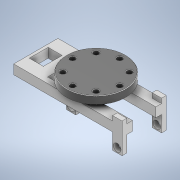
# Autodesk Inventor part: KukaHead
Saved by Autodesk Inventor 2021 (Build 250183000, 183)
## iProperties
Created: 2021-06-08
Part Number: KukaHead
Material: Generic
Document SubType Name: Modeling
Designer: zmac845
Density: 1 g/cm^3
Appearance: Default
Author: zmac845
Autodesk Inventor part; units mm, degrees
ref_plane "YZ Plane" through (0, 0, 0) normal (1, 0, 0) x (0, 1, 0)
ref_plane "XZ Plane" through (0, 0, 0) normal (0, 1, 0) x (-1, 0, 0)
ref_plane "XY Plane" through (0, 0, 0) normal (0, 0, 1) x (1, 0, 0)
sketch "Sketch1" plane through (0, 0, 0) normal (0, 1, 0) x (-1, 0, 0)
  circle A0 centre (0, 0) radius 31.25
  circle A1 centre (0, 25) radius 2.75
  circle A2 centre (-17.6777, 17.6777) radius 2.75
  circle A3 centre (-25, 0) radius 2.75
  circle A4 centre (-17.6777, -17.6777) radius 2.75
  circle A5 centre (0, -25) radius 2.75
  circle A6 centre (17.6777, -17.6777) radius 2.75
  circle A7 centre (25, 0) radius 2.75
  circle A8 centre (17.6777, 17.6777) radius 2.75
  dimension "d0" = 62.5
  dimension "d2" = 5.5
  dimension "d3" = 25
  dimension "d6" = 360
  constraints: 9 centre point, 1 coincident, 1 vertical alignment, 17 other
  measures "d0" diameter of A0
  measures "d2" diameter of A1
  measures "d3" distance of point (0, 0) A1.centre
extrude "Extrusion1" add sketch "Sketch1" along normal blind 8
fillet "Fillet1" radius 0.5 9 edges at (31.25, 8, 0) (-22.25, 8, 0) (-14.9277, 8, 17.6777) (-14.9277, 8, -17.6777) (2.75, 8, -25) (20.4277, 8, -17.6777) (27.75, 8, 0) (20.4277, 8, 17.6777) (2.75, 8, 25)
sketch "Sketch8" plane through (0, 0, 0) normal (0, -1, 0) x (1, 0, 0)
  line L0 (-35, 35) -> (-35, -35) projected
  line L1 (-35, 0) -> (-35, 12.5)
  line L2 (-35, 12.5) -> (-14, 12.5)
  line L3 (-14, 12.5) -> (-4, 12.5)
  line L4 (-4, 12.5) -> (-4, 17.5)
  line L5 (-4, 17.5) -> (-14, 17.5)
  line L6 (-14, 17.5) -> (-14, 12.5)
  line L7 (-35, 0) -> (-35, -12.5)
  line L8 (-35, -12.5) -> (-14, -12.5)
  line L9 (-14, -12.5) -> (-4, -12.5)
  line L10 (-4, -12.5) -> (-4, -17.5)
  line L11 (-4, -17.5) -> (-14, -17.5)
  line L12 (-14, -17.5) -> (-14, -12.5)
  point P0 (0, 0)
  dimension "d27" = 12.5
  dimension "d28" = 21
  dimension "d29" = 10
  dimension "d30" = 5
  dimension "d31" = 12.5
  dimension "d32" = 21
  dimension "d33" = 10
  dimension "d34" = 5
  constraints: 24 end point, 7 point on line, 5 perpendicular, 1 midpoint
  measures "d27" distance of L1.start L1.end
  measures "d28" distance of L1.end L2.end
  measures "d29" distance of L2.end L3.end
  measures "d30" distance of L3.end L4.end
  measures "d31" distance of L1.start L7.end
  measures "d32" distance of L7.end L8.end
  measures "d33" distance of L8.end L9.end
  measures "d34" distance of L9.end L10.end
extrude "Extrusion5" add sketch "Sketch8" along normal blind 25
sketch "Sketch9" plane through (0, 0, 0) normal (0, -1, 0) x (1, 0, 0)
  line L0 (-4, 12.5) -> (-14, 12.5) projected
  line L1 (-9, 12.5) -> (41, 12.5)
  line L2 (41, 12.5) -> (41, 17.5)
  line L3 (41, 17.5) -> (51, 17.5)
  line L4 (51, 17.5) -> (51, 12.5)
  line L5 (51, 12.5) -> (41, 12.5)
  line L6 (-14, -17.5) -> (-4, -17.5) projected
  line L7 (-9, -17.5) -> (41, -17.5)
  line L8 (41, -17.5) -> (51, -17.5)
  line L9 (51, -17.5) -> (51, -12.5)
  line L10 (51, -12.5) -> (41, -12.5)
  line L11 (41, -12.5) -> (41, -17.5)
  line L12 (41, 12.5) -> (41, 18.5)
  line L13 (41, 18.5) -> (51, 18.5)
  line L14 (51, 18.5) -> (51, 23.5)
  line L15 (51, 23.5) -> (41, 23.5)
  line L16 (41, 23.5) -> (41, 18.5)
  line L17 (41, -12.5) -> (41, -18.5)
  line L18 (41, -18.5) -> (51, -18.5)
  line L19 (51, -18.5) -> (51, -23.5)
  line L20 (51, -23.5) -> (41, -23.5)
  line L21 (41, -23.5) -> (41, -18.5)
  point P0 (0, 0)
  dimension "d37" = 50
  dimension "d38" = 5
  dimension "d39" = 10
  dimension "d40" = 50
  dimension "d41" = 5
  dimension "d42" = 6
  dimension "d43" = 5
  dimension "d44" = 6
  dimension "d45" = 10
  dimension "d46" = 5
  constraints: 40 end point, 14 perpendicular, 5 point on line, 2 collinear, 2 midpoint, 1 horizontal
  measures "d37" distance of L1.start L1.end
  measures "d38" distance of L1.end L2.end
  measures "d39" distance of L2.end L3.end
  measures "d40" distance of L7.start L7.end
  measures "d41" distance of L8.end L9.end
  measures "d42" distance of L1.end L12.end
  measures "d43" distance of L13.end L14.end
  measures "d44" distance of L10.end L17.end
  measures "d45" distance of L17.end L18.end
  measures "d46" distance of L18.end L19.end
sketch "Sketch10" plane through (-14, 0, 17.5) normal (0, 0, 1) x (1, 0, 0)
  point P0 (14, 0)
sketch "Sketch11" plane through (-14, 0, 17.5) normal (0, 0, 1) x (1, 0, 0)
  point P0 (14, 0)
sketch "Sketch12" plane through (0, -25, 0) normal (0, -1, 0) x (1, 0, 0)
  point P0 (0, 0)
sketch "Sketch13" plane through (-14, 0, 17.5) normal (0, 0, 1) x (1, 0, 0)
  line L0 (10, -25) -> (0, -25) projected
  line L1 (5, -25) -> (5, -20)
  circle A0 centre (5, -20) radius 4
  point P0 (14, 0)
  dimension "d49" = 5
  dimension "d50" = 8
  constraints: 2 end point, 1 centre point, 1 coincident, 1 midpoint, 1 vertical
  measures "d49" distance of L1.start L1.end
  measures "d50" diameter of A0
extrude "Extrusion7" cut sketch "Sketch13" against normal blind 40
sketch "Sketch14" plane through (-14, 0, 17.5) normal (0, 0, 1) x (1, 0, 0)
  point P0 (14, 0)
extrude "Extrusion8" add sketch "Sketch9" along normal blind 32 contours L16 L15 L14 L13 | L18 L19 L20 L21
sketch "Sketch18" plane through (41, 0, 23.5) normal (0, 0, 1) x (1, 0, 0)
  line L0 (0, -32) -> (10, -32) projected
  line L1 (5, -32) -> (5, -27)
  circle A0 centre (5, -27) radius 4
  point P0 (-41, 0)
  dimension "d55" = 5
  dimension "d56" = 8
  constraints: 2 end point, 1 centre point, 1 coincident, 1 midpoint, 1 vertical
  measures "d55" distance of L1.start L1.end
  measures "d56" diameter of A0
extrude "Extrusion9" cut sketch "Sketch18" against normal blind 60
sketch "Sketch19" plane through (41, 0, 23.5) normal (0, 0, 1) x (1, 0, 0)
  point P0 (-41, 0)
sketch "Sketch20" plane through (0, -25, 0) normal (0, -1, 0) x (1, 0, 0)
  point P0 (0, 0)
sketch "Sketch21" plane through (-14, 0, 17.5) normal (0, 0, 1) x (1, 0, 0)
  point P0 (14, 0)
sketch "Sketch22" plane through (-14, 0, 12.5) normal (-1, 0, 0) x (0, 0, 1)
  line L0 (0, 0) -> (0, -25) projected
  line L1 (0, 0) -> (0, -5)
  line L2 (0, -5) -> (11, -5)
  line L3 (11, 0) -> (11, -32) projected
  line L4 (11, -5) -> (11, -15)
  line L5 (11, -15) -> (0, -15)
  line L6 (0, -5) -> (0, -15)
  point P0 (-12.5, 0)
  dimension "d59" = 5
  dimension "d60" = 10
  constraints: 10 end point, 4 point on line, 2 perpendicular, 1 collinear
  measures "d59" distance of L0.start L1.end
  measures "d60" distance of L2.end L4.end
extrude "Extrusion10" add sketch "Sketch22" against normal blind 65
sketch "Sketch23" plane through (-14, 0, -17.5) normal (-1, 0, 0) x (0, 0, 1)
  line L0 (5, 0) -> (5, -25) projected
  line L1 (5, 0) -> (5, -5)
  line L2 (5, -5) -> (-6, -5)
  line L3 (-6, 0) -> (-6, -32) projected
  line L4 (-6, -5) -> (-6, -15)
  line L5 (-6, -15) -> (5, -15)
  line L6 (5, -5) -> (5, -15)
  point P0 (17.5, 0)
  dimension "d63" = 5
  dimension "d64" = 10
  constraints: 10 end point, 4 point on line, 3 perpendicular
  measures "d63" distance of L0.start L1.end
  measures "d64" distance of L2.end L4.end
extrude "Extrusion11" add sketch "Sketch23" against normal blind 65
sketch "Sketch24" plane through (51, -32, 18.5) normal (0, 0, -1) x (-1, 0, 0)
  point P0 (51, 32)
sketch "Sketch25" plane through (-14, 0, -17.5) normal (-1, 0, 0) x (0, 0, 1)
  point P0 (17.5, 0)
sketch "Sketch26" plane through (-14, 0, -17.5) normal (-1, 0, 0) x (0, 0, 1)
  point P0 (17.5, 0)
sketch "Sketch27" plane through (-14, 0, -17.5) normal (-1, 0, 0) x (0, 0, 1)
  line L0 (0, -5) -> (-6, -5) projected
  line L1 (-6, -5) -> (0, -5)
  line L2 (-6, -15) -> (0, -15) projected
  line L3 (0, -5) -> (0, -15)
  line L4 (0, -15) -> (-6, -15)
  line L5 (-6, -15) -> (-6, -5)
  point P0 (17.5, 0)
  constraints: 8 end point, 2 collinear, 2 perpendicular
extrude "Extrusion12" add sketch "Sketch27" along normal blind 55
sketch "Sketch28" plane through (-14, 0, 12.5) normal (-1, 0, 0) x (0, 0, 1)
  line L0 (11, -5) -> (5, -5) projected
  line L1 (5, -5) -> (11, -5)
  line L2 (11, -15) -> (11, -32) projected
  line L3 (11, -5) -> (11, -15)
  line L4 (5, -15) -> (11, -15) projected
  line L5 (11, -15) -> (5, -15)
  line L6 (5, -15) -> (5, -5)
  point P0 (-12.5, 0)
  constraints: 8 end point, 2 collinear, 2 perpendicular
extrude "Extrusion13" add sketch "Sketch28" along normal blind 55
sketch "Sketch29" plane through (-4, -5, -12.5) normal (0, 1, 0) x (1, 0, 0)
  line L0 (45, 11) -> (-65, 11) projected
  line L1 (-65, -36) -> (45, -36) projected
  line L2 (-65, 11) -> (-65, -36)
  line L3 (-65, -36) -> (-30, -36)
  line L4 (-30, -36) -> (-30, 11)
  line L5 (-65, 11) -> (-30, 11)
  point P0 (4, -12.5)
  dimension "d71" = 35
  constraints: 8 end point, 2 point on line, 1 collinear, 1 perpendicular, 1 vertical
  measures "d71" distance of L1.start L3.end
extrude "Extrusion14" add sketch "Sketch29" against normal blind 10
sketch "Sketch30" plane through (-4, -5, 12.5) normal (0, 1, 0) x (1, 0, 0)
  point P0 (4, 12.5)
sketch "Sketch31" plane through (-4, -15, 12.5) normal (0, -1, 0) x (1, 0, 0)
  line L0 (-65, 11) -> (-65, -36) projected
  line L1 (-65, 11) -> (-60, 11)
  line L2 (-65, 11) -> (45, 11) projected
  line L3 (-60, 11) -> (-60, -36)
  line L4 (45, -36) -> (-65, -36) projected
  line L5 (-65, -36) -> (-65, 11)
  point P0 (4, -12.5)
  dimension "d74" = 5
  constraints: 6 end point, 2 point on line, 1 parallel, 1 perpendicular
  measures "d74" distance of L0.start L1.end
extrude "Extrusion15" cut sketch "Sketch31" against normal blind 35
sketch "Sketch32" plane through (-4, -15, -12.5) normal (0, -1, 0) x (1, 0, 0)
  line L0 (-30, 30) -> (-30, -5) projected
  line L1 (-30, 12.5) -> (-57, 12.5)
  line L2 (-57, 12.5) -> (-57, 22.5)
  line L3 (-57, 22.5) -> (-42, 22.5)
  line L4 (-42, 22.5) -> (-42, 2.5)
  line L5 (-42, 2.5) -> (-57, 2.5)
  line L6 (-57, 2.5) -> (-57, 12.5)
  point P0 (4, 12.5)
  dimension "d77" = 27
  dimension "d78" = 10
  dimension "d79" = 15
  dimension "d80" = 20
  constraints: 12 end point, 5 perpendicular, 1 horizontal, 1 midpoint, 1 point on line
  measures "d77" distance of L1.start L1.end
  measures "d78" distance of L1.end L2.end
  measures "d79" distance of L2.end L3.end
  measures "d80" distance of L3.end L4.end
extrude "Extrusion16" cut sketch "Sketch32" against normal blind 35
body "Solid1"
